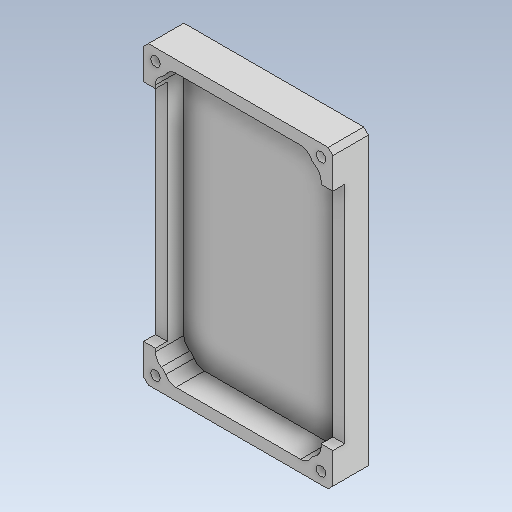
# Autodesk Inventor part: 0008-10-049 Capac Mofset
Saved by Autodesk Inventor 2020 (Build 240168000, 168)
## iProperties
Created: 2020-03-06
Part Number: 0008-10-049 Capac Mofset
Material: Generic
Document SubType Name: Modeling
Designer: 40743
Density: 1 g/cm^3
Appearance: Default
Description: Capac mofset
Mass: 48.912 g
Surface Area: 291.541 cm^2
Volume: 48.912 cm^3
Author: 40743
Subject: 049
Autodesk Inventor part; units mm, degrees
ref_plane "YZ Plane" through (0, 0, 0) normal (1, 0, 0) x (0, 1, 0)
ref_plane "XZ Plane" through (0, 0, 0) normal (0, 1, 0) x (-1, 0, 0)
ref_plane "XY Plane" through (0, 0, 0) normal (0, 0, 1) x (1, 0, 0)
sketch "Sketch1" plane through (0, 0, 0) normal (0, 0, 1) x (1, 0, 0)
  line L0 (-40, 62.5) -> (40, 62.5)
  line L1 (40, 62.5) -> (40, -62.5)
  line L2 (40, -62.5) -> (-40, -62.5)
  line L3 (-40, -62.5) -> (-40, 62.5)
  point P0 (0, 0)
  point P1 (0, 62.5)
  point P2 (-40, 0)
  dimension "d0" = 80
  dimension "d1" = 125
  constraints: 8 end point, 2 midpoint, 2 parallel, 1 horizontal, 1 horizontal alignment, 1 perpendicular, 1 vertical alignment
  measures "d0" distance of L0.start L0.end
  measures "d1" distance of L2.end L0.start
extrude "Extrusion1" add sketch "Sketch1" along normal blind 15
sketch "Sketch2" plane through (0, 0, 15) normal (0, 0, 1) x (1, 0, 0)
  line L0 (40, 62.5) -> (-40, 62.5) projected
  line L1 (-40, 62.5) -> (-40, -62.5) projected
  line L2 (-40, -62.5) -> (40, -62.5) projected
  line L3 (40, -62.5) -> (40, 62.5) projected
  line L4 (35, 57.5) -> (-35, 57.5)
  line L5 (-35, 57.5) -> (-35, -57.5)
  line L6 (-35, -57.5) -> (35, -57.5)
  line L7 (35, -57.5) -> (35, 57.5)
  point P0 (0, 0)
  dimension "d4" = 5
  constraints: 8 end point, 3 other
  measures "d4" distance between parallel lines of L7 L3
extrude "Extrusion2" cut sketch "Sketch2" against normal blind 12 contours L7 L6 L5 L4
sketch "Sketch3" plane through (0, 0, 0) normal (0, 0, -1) x (-1, 0, 0)
  line L0 (-35, -57.5) -> (35, -57.5) construction
  line L1 (35, -57.5) -> (35, 57.5) construction
  line L2 (35, 57.5) -> (-35, 57.5) construction
  line L3 (-35, 57.5) -> (-35, -57.5) construction
  line L4 (-40, 62.5) -> (40, 62.5) construction
  line L5 (-40, -62.5) -> (-40, 62.5) construction
  line L6 (40, -62.5) -> (-40, -62.5) construction
  line L7 (-35, 57.5) -> (-35, -57.5) projected
  line L8 (35, 57.5) -> (-35, 57.5) projected
  line L9 (35, -57.5) -> (35, 57.5) projected
  line L10 (-35, -57.5) -> (35, -57.5) projected
  point P0 (0, 0)
  point P1 (0, 57.5)
  point P2 (0, 62.5)
  point P3 (-35, 0)
  point P4 (-40, 0)
  dimension "d27" = 115
  dimension "d28" = 70
  constraints: 8 end point, 4 coincident, 4 midpoint, 2 parallel, 1 horizontal, 1 horizontal alignment, 1 perpendicular, 1 vertical alignment
  measures "d27" distance of L0.end L1.end
  measures "d28" distance of L1.end L2.end
hole "Hole1" at (35, -57.5, 0) at (35, 57.5, 0) at (-35, 57.5, 0) at (-35, -57.5, 0) direction (0, 0, 1) diameter 4 end through all
sketch "Sketch4" plane through (0, 0, 3) normal (0, 0, 1) x (1, 0, 0)
  circle A0 centre (35, -57.5) radius 5
  circle A1 centre (35, 57.5) radius 5
  circle A2 centre (-35, 57.5) radius 5
  circle A3 centre (-35, -57.5) radius 5
  arc A4 (35, -55.5) -> (33, -57.5) centre (35, -57.5) ccw projected
  arc A5 (-33, -57.5) -> (-35, -55.5) centre (-35, -57.5) ccw projected
  arc A6 (-35, 55.5) -> (-33, 57.5) centre (-35, 57.5) ccw projected
  arc A7 (33, 57.5) -> (35, 55.5) centre (35, 57.5) ccw projected
  circle A8 centre (35, 57.5) radius 2 projected
  circle A9 centre (35, 57.5) radius 2
  circle A10 centre (35, -57.5) radius 2
  circle A11 centre (-35, -57.5) radius 2
  circle A12 centre (-35, 57.5) radius 2
  point P0 (0, 0)
  point P1 (37, -57.5)
  point P2 (-35, -59.5)
  point P3 (-37, 57.5)
  point P4 (35, 59.5)
  point P5 (-35, -59.5)
  point P6 (-35, -55.5)
  point P7 (35, -55.5)
  point P8 (-37, 57.5)
  dimension "d16" = 10
  constraints: 6 centre point, 5 concentric, 4 coincident, 3 equal radius, 6 other
  measures "d16" diameter of A0
extrude "Extrusion3" add sketch "Sketch4" along normal up to surface (12 mm away)
fillet "Fillet1" radius 5 8 edges at (-35, -52.5, 9) (-30, -57.5, 9) (-35, 52.5, 9) (-30, 57.5, 9) (35, 52.5, 9) (30, 57.5, 9) (30, -57.5, 9) (35, -52.5, 9)
sketch "Sketch6" plane through (0, 0, 0) normal (1, 0, 0) x (0, 1, 0)
  line L0 (47.4997, 10) -> (-47.4997, 10)
  line L1 (-47.4997, 10) -> (-47.4997, 15)
  line L2 (-47.4997, 15) -> (47.4997, 15)
  line L3 (47.4997, 15) -> (47.4997, 10)
  line L4 (-62.5, 0) -> (62.5, 0) projected
  line L5 (-57.5, 15) -> (57.5, 15) projected
  line L6 (-48.8397, 15) -> (-48.8397, 3) projected
  line L7 (48.8397, 3) -> (48.8397, 15) projected
  point P0 (0, 0)
  dimension "d32" = 5
  dimension "d33" = 1.34
  dimension "d34" = 1.34
  constraints: 8 end point, 2 parallel, 1 collinear, 1 horizontal, 1 perpendicular
  measures "d32" distance between parallel lines of L0 L2
  measures "d33" distance between parallel lines of L6 L1
  measures "d34" distance between parallel lines of L3 L7
extrude "Extrusion5" cut sketch "Sketch6" against normal through all both and the other way through all
chamfer "Chamfer1" distance 2 angle 45 4 edges at (40, 62.5, 7.5) (-40, 62.5, 7.5) (40, -62.5, 7.5) (-40, -62.5, 7.5)
equation "\"d34\" = d33"
body "Solid1"
